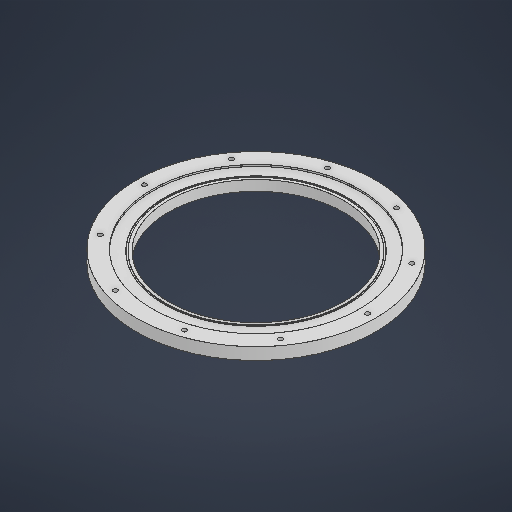
# Autodesk Inventor part: 260mm housing 2
Saved by Autodesk Inventor 2025 (Build 290162000, 162)
## iProperties
Created: 2024-10-30
Part Number: 260mm housing 2
Material: Generic
Document SubType Name: Modeling
Designer: mayhe
Density: 1 g/cm^3
Appearance: Default
Author: mayhe
Autodesk Inventor part; units mm, degrees
ref_plane "YZ Plane" through (0, 0, 0) normal (1, 0, 0) x (0, 1, 0)
ref_plane "XZ Plane" through (0, 0, 0) normal (0, 1, 0) x (-1, 0, 0)
ref_plane "XY Plane" through (0, 0, 0) normal (0, 0, 1) x (1, 0, 0)
sketch "Sketch1" plane through (0, 0, 0) normal (0, 1, 0) x (-1, 0, 0)
  circle A0 centre (0, 0) radius 150
  circle A1 centre (0, 0) radius 110
  circle A2 centre (0, 0) radius 125
  circle A3 centre (0, 0) radius 140
  circle A4 centre (0, 125) radius 2.75
  line L0 (-4.0625, 127.3455) -> (0, 129.691)
  line L1 (0, 129.691) -> (4.0625, 127.3455)
  line L2 (4.0625, 127.3455) -> (4.0625, 122.6545)
  line L3 (4.0625, 122.6545) -> (0, 120.309)
  line L4 (0, 120.309) -> (-4.0625, 122.6545)
  line L5 (-4.0625, 122.6545) -> (-4.0625, 127.3455)
  circle A5 centre (-73.4732, 101.1271) radius 2.75
  line L6 (-78.1384, 100.6368) -> (-76.2304, 104.9222)
  line L7 (-76.2304, 104.9222) -> (-71.5652, 105.4125)
  line L8 (-71.5652, 105.4125) -> (-68.8079, 101.6175)
  line L9 (-68.8079, 101.6175) -> (-70.7159, 97.332)
  line L10 (-70.7159, 97.332) -> (-75.3811, 96.8417)
  line L11 (-75.3811, 96.8417) -> (-78.1384, 100.6368)
  circle A6 centre (-118.8821, 38.6271) radius 2.75
  line L12 (-122.3681, 35.4883) -> (-123.3434, 40.0767)
  line L13 (-123.3434, 40.0767) -> (-119.8574, 43.2156)
  line L14 (-119.8574, 43.2156) -> (-115.396, 41.766)
  line L15 (-115.396, 41.766) -> (-114.4207, 37.1775)
  line L16 (-114.4207, 37.1775) -> (-117.9068, 34.0387)
  line L17 (-117.9068, 34.0387) -> (-122.3681, 35.4883)
  circle A7 centre (-118.8821, -38.6271) radius 2.75
  line L18 (-119.8574, -43.2156) -> (-123.3434, -40.0767)
  line L19 (-123.3434, -40.0767) -> (-122.3681, -35.4883)
  line L20 (-122.3681, -35.4883) -> (-117.9068, -34.0387)
  line L21 (-117.9068, -34.0387) -> (-114.4207, -37.1775)
  line L22 (-114.4207, -37.1775) -> (-115.396, -41.766)
  line L23 (-115.396, -41.766) -> (-119.8574, -43.2156)
  circle A8 centre (-73.4732, -101.1271) radius 2.75
  line L24 (-71.5652, -105.4125) -> (-76.2304, -104.9222)
  line L25 (-76.2304, -104.9222) -> (-78.1384, -100.6368)
  line L26 (-78.1384, -100.6368) -> (-75.3811, -96.8417)
  line L27 (-75.3811, -96.8417) -> (-70.7159, -97.332)
  line L28 (-70.7159, -97.332) -> (-68.8079, -101.6175)
  line L29 (-68.8079, -101.6175) -> (-71.5652, -105.4125)
  circle A9 centre (0, -125) radius 2.75
  line L30 (4.0625, -127.3455) -> (0, -129.691)
  line L31 (0, -129.691) -> (-4.0625, -127.3455)
  line L32 (-4.0625, -127.3455) -> (-4.0625, -122.6545)
  line L33 (-4.0625, -122.6545) -> (0, -120.309)
  line L34 (0, -120.309) -> (4.0625, -122.6545)
  line L35 (4.0625, -122.6545) -> (4.0625, -127.3455)
  circle A10 centre (73.4732, -101.1271) radius 2.75
  line L36 (78.1384, -100.6368) -> (76.2304, -104.9222)
  line L37 (76.2304, -104.9222) -> (71.5652, -105.4125)
  line L38 (71.5652, -105.4125) -> (68.8079, -101.6175)
  line L39 (68.8079, -101.6175) -> (70.7159, -97.332)
  line L40 (70.7159, -97.332) -> (75.3811, -96.8417)
  line L41 (75.3811, -96.8417) -> (78.1384, -100.6368)
  circle A11 centre (118.8821, -38.6271) radius 2.75
  line L42 (122.3681, -35.4883) -> (123.3434, -40.0767)
  line L43 (123.3434, -40.0767) -> (119.8574, -43.2156)
  line L44 (119.8574, -43.2156) -> (115.396, -41.766)
  line L45 (115.396, -41.766) -> (114.4207, -37.1775)
  line L46 (114.4207, -37.1775) -> (117.9068, -34.0387)
  line L47 (117.9068, -34.0387) -> (122.3681, -35.4883)
  circle A12 centre (118.8821, 38.6271) radius 2.75
  line L48 (119.8574, 43.2156) -> (123.3434, 40.0767)
  line L49 (123.3434, 40.0767) -> (122.3681, 35.4883)
  line L50 (122.3681, 35.4883) -> (117.9068, 34.0387)
  line L51 (117.9068, 34.0387) -> (114.4207, 37.1775)
  line L52 (114.4207, 37.1775) -> (115.396, 41.766)
  line L53 (115.396, 41.766) -> (119.8574, 43.2156)
  circle A13 centre (73.4732, 101.1271) radius 2.75
  line L54 (71.5652, 105.4125) -> (76.2304, 104.9222)
  line L55 (76.2304, 104.9222) -> (78.1384, 100.6368)
  line L56 (78.1384, 100.6368) -> (75.3811, 96.8417)
  line L57 (75.3811, 96.8417) -> (70.7159, 97.332)
  line L58 (70.7159, 97.332) -> (68.8079, 101.6175)
  line L59 (68.8079, 101.6175) -> (71.5652, 105.4125)
  point P0 (-4.0625, 125)
  point P1 (-76.7598, 98.7392)
  point P2 (-120.1374, 34.7635)
  point P3 (-117.6267, -42.4908)
  point P4 (-70.1865, -103.515)
  point P5 (4.0625, -125)
  point P6 (76.7598, -98.7392)
  point P7 (120.1374, -34.7635)
  point P8 (117.6267, 42.4908)
  point P9 (70.1865, 103.515)
  dimension "d2" = 250
  dimension "d0" = 300
  dimension "d1" = 220
  dimension "d4" = 280
  dimension "d7" = 5.5
  dimension "d11" = 360
  constraints: 120 end point, 13 centre point, 5 coincident, 1 midpoint, 1 vertical alignment, 176 other
  measures "d0" diameter of A0
  measures "d1" diameter of A1
  measures "d4" diameter of A3
  measures "d7" diameter of A4
extrude "Extrusion1" add sketch "Sketch1" along normal blind 2 contours A0 | A2 L47 L46 L45 L44 L41 L40 L39 L38 L35 L34 L33 L32 L29 L28 L27 L26 L23 L22 L21 L20 L17 L16 L15 L14 L11 L10 L9 L8 L5 L4 L3 L2 L59 L58 L57 L56 L53 L52 L51 L50 | L50 L51 L52 L53 A2 A12 | A2 A12 L53 L48 L49 L50 | L47 L42 L43 L44 A2 A11 | A2 A11 L44 L45 L46 L47 | L56 L57 L58 L59 A2 A13 | A2 A13 L59 L54 L55 L56 | L41 L36 L37 L38 A2 A10 | A2 A10 L38 L39 L40 L41 | L2 L3 L4 L5 A2 A4 | A2 A4 L5 L0 L1 L2 | L35 L30 L31 L32 A2 A9 | A2 A9 L32 L33 L34 L35 | L8 L9 L10 L11 A2 A5 | A2 A5 L11 L6 L7 L8 | L29 L24 L25 L26 A2 A8 | A2 A8 L26 L27 L28 L29 | L14 L15 L16 L17 A2 A6 | A2 A6 L17 L12 L13 L14 | L23 L18 L19 L20 A2 A7 | A2 A7 L20 L21 L22 L23 | A3
sketch "Sketch2" plane through (0, 2, 0) normal (0, 1, 0) x (1, 0, 0)
  point P0 (0, 0)
extrude "Extrusion2" add sketch "Sketch1" along normal blind 6.25 contours A0 | A2 L47 L46 L45 L44 L41 L40 L39 L38 L35 L34 L33 L32 L29 L28 L27 L26 L23 L22 L21 L20 L17 L16 L15 L14 L11 L10 L9 L8 L5 L4 L3 L2 L59 L58 L57 L56 L53 L52 L51 L50 | A3
sketch "Sketch3" plane through (0, 6.25, 0) normal (0, 1, 0) x (1, 0, 0)
  circle A0 centre (0, 0) radius 110
  circle A1 centre (0, 0) radius 150
  circle A2 centre (0, 125) radius 2.75 projected
  circle A3 centre (0, 0) radius 125
  circle A4 centre (0, 125) radius 2.75
  circle A5 centre (-73.4732, 101.1271) radius 2.75
  circle A6 centre (-118.8821, 38.6271) radius 2.75
  circle A7 centre (-118.8821, -38.6271) radius 2.75
  circle A8 centre (-73.4732, -101.1271) radius 2.75
  circle A9 centre (0, -125) radius 2.75
  circle A10 centre (73.4732, -101.1271) radius 2.75
  circle A11 centre (118.8821, -38.6271) radius 2.75
  circle A12 centre (118.8821, 38.6271) radius 2.75
  circle A13 centre (73.4732, 101.1271) radius 2.75
  dimension "d15" = 250
  dimension "d18" = 360
  constraints: 12 centre point, 4 coincident, 1 concentric, 1 vertical alignment, 23 other
extrude "Extrusion3" add sketch "Sketch3" along normal blind 4.75 contours A1 | A2 A3 A13 A12 A11 A10 A9 A8 A7 A6 A5
sketch "Sketch5" plane through (0, 11, 0) normal (0, 1, 0) x (1, 0, 0)
  circle A0 centre (0, 0) radius 110
  circle A1 centre (0, 0) radius 150
  constraints: 2 centre point, 2 coincident
extrude "Extrusion6" add sketch "Sketch5" along normal blind 4
sketch "Sketch6" plane through (0, 15, 0) normal (0, 1, 0) x (1, 0, 0)
  circle A0 centre (0, 0) radius 130
  dimension "d29" = 260
  constraints: 1 centre point, 1 coincident
  measures "d29" diameter of A0
extrude "Extrusion7" cut sketch "Sketch6" against normal blind 2.125
sketch "Sketch8" plane through (0, 0, 0) normal (0, -1, 0) x (1, 0, 0)
  circle A0 centre (0, 0) radius 140
  circle A1 centre (140, 0) radius 2.75
  circle A2 centre (113.2624, 82.2899) radius 2.75
  circle A3 centre (43.2624, 133.1479) radius 2.75
  circle A4 centre (-43.2624, 133.1479) radius 2.75
  circle A5 centre (-113.2624, 82.2899) radius 2.75
  circle A6 centre (-140, 0) radius 2.75
  circle A7 centre (-113.2624, -82.2899) radius 2.75
  circle A8 centre (-43.2624, -133.1479) radius 2.75
  circle A9 centre (43.2624, -133.1479) radius 2.75
  circle A10 centre (113.2624, -82.2899) radius 2.75
  dimension "d45" = 280
  dimension "d46" = 5.5
  dimension "d49" = 360
  constraints: 10 centre point, 1 coincident, 1 horizontal alignment, 23 other
  measures "d46" diameter of A1
hole "Hole2" at (-43.2624, 0, -133.1479) at (-113.2624, 0, -82.2899) at (-140, 0, 0) at (-113.2624, 0, 82.2899) at (-43.2624, 0, 133.1479) at (43.2624, 0, 133.1479) at (113.2624, 0, 82.2899) at (140, 0, 0) at (113.2624, 0, -82.2899) at (43.2624, 0, -133.1479) direction (0, 1, 0) diameter 5.5 end through all counterbore diameter 10.475 counterbore depth 7.375
sketch "Sketch9" plane through (0, 0, 0) normal (1, 0, 0) x (0, 1, 0)
  line L0 (12.875, -110) -> (12.875, 110) projected
  line L1 (12.875, -110) -> (0, -110)
  line L2 (12.875, -110) -> (0, -110) projected
  line L3 (13.875, -115.5) -> (11.875, -115.5)
  line L4 (11.875, -115.5) -> (11.875, -113.5)
  line L5 (11.875, -113.5) -> (13.875, -113.5)
  line L6 (13.875, -113.5) -> (13.875, -115.5)
  line L7 (12.875, 130) -> (12.875, -130) projected
  line L8 (13.875, -115.5) -> (11.875, -113.5) construction
  line L9 (11.875, -115.5) -> (13.875, -113.5) construction
  line L10 (1, -115.5) -> (-1, -115.5)
  line L11 (-1, -115.5) -> (-1, -113.5)
  line L12 (-1, -113.5) -> (1, -113.5)
  line L13 (1, -113.5) -> (1, -115.5)
  line L14 (0, -150) -> (0, 150) projected
  line L15 (1, -115.5) -> (-1, -113.5) construction
  line L16 (-1, -115.5) -> (1, -113.5) construction
  line L17 (-4.2, 0) -> (18.2, 0) projected
  point P0 (0, 0)
  point P1 (12.875, -114.5)
  point P2 (0, -114.5)
  dimension "d58" = 2
  dimension "d59" = 2
  dimension "d60" = 4.5
  dimension "d61" = 2
  dimension "d62" = 2
  constraints: 26 end point, 4 midpoint, 4 parallel, 3 point on line, 2 horizontal, 2 perpendicular
  measures "d58" distance of L4.end L5.end
  measures "d59" distance of L3.end L4.end
  measures "d60" distance from line of L1 point (12.875, -114.5)
  measures "d61" distance of L11.end L12.end
  measures "d62" distance of L10.end L11.end
revolve "Revolution1" cut sketch "Sketch9" angle 360 about axis through (0, -10, 0) along (0, 1, 0) contours L3 L7 L5 L6 | L3 L4 L5 L7 | L10 L14 L12 L13 | L10 L11 L12 L14
body "Solid1"
